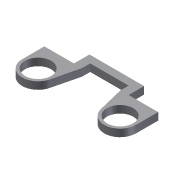
# Autodesk Inventor part: Suporte - Baterias
Saved by Autodesk Inventor 2011 (Build 150239000, 239)
## iProperties
Created: 2011-04-09
Part Number: Suporte - Baterias
Document SubType Name: Modeling
Designer: Milton
Density: 1 g/cm^3
Author: Milton
Autodesk Inventor part; units mm, degrees
ref_plane "YZ Plane" through (0, 0, 0) normal (1, 0, 0) x (0, 1, 0)
ref_plane "XZ Plane" through (0, 0, 0) normal (0, 1, 0) x (-1, 0, 0)
ref_plane "XY Plane" through (0, 0, 0) normal (0, 0, 1) x (1, 0, 0)
sketch "Sketch1" plane through (0, 0, 0) normal (0, 0, 1) x (1, 0, 0)
  line L0 (38.75, 17.7481) -> (-13.25, 17.75)
  circle A0 centre (68.25, -23.2519) radius 17.75
  circle A1 centre (-42.75, -23.2512) radius 17.75
  circle A2 centre (68.25, -23.2519) radius 21.5
  circle A3 centre (-42.75, -23.2512) radius 21.5
  line L1 (49.75, 27.75) -> (-24.25, 27.75)
  line L2 (-24.25, 6.7504) -> (-74.75, 6.7484)
  line L3 (49.75, 27.75) -> (49.75, 6.7488)
  line L4 (38.75, 17.7481) -> (38.75, 6.7503)
  line L5 (-13.25, 17.75) -> (-13.25, 6.7503)
  line L6 (-24.25, 27.75) -> (-24.25, 6.7504)
  line L7 (38.75, 6.7503) -> (47.3695, -28.3757)
  line L8 (-13.25, 6.7503) -> (-21.8695, -28.3751)
  line L9 (-74.75, 6.7503) -> (-74.75, -44.7512)
  line L10 (-42.75, -44.7512) -> (-74.75, -44.7512)
  line L11 (68.25, -44.7519) -> (100.25, -44.7519)
  line L12 (100.25, -44.7519) -> (100.25, 6.7488)
  line L13 (49.75, 6.7488) -> (100.25, 6.7488)
  point P0 (0, 0)
  point P1 (-64.25, -23.2512)
  point P2 (89.75, -23.2512)
  dimension "d6" = 35.5
  dimension "d7" = 35.5
  dimension "d14" = 43
  dimension "d15" = 43
  dimension "d23" = 52
  dimension "d25" = 11
  dimension "d26" = 11
  dimension "d29" = 29.5
  dimension "d30" = 29.5
  dimension "d31" = 32
  dimension "d32" = 32
  constraints: 28 end point, 6 point on circle, 4 centre point, 4 parallel, 4 tangent, 3 perpendicular, 2 coincident, 1 point on line
  measures "d6" diameter of A0
  measures "d7" diameter of A1
  measures "d14" diameter of A2
  measures "d15" diameter of A3
  measures "d23" distance of L0.start L0.end
  measures "d25" distance between parallel lines of L3 L4
  measures "d26" distance between parallel lines of L6 L5
  measures "d29" distance from line of L4 A0.centre
  measures "d30" distance from line of A1.centre L5
  measures "d31" distance from line of L12 A2.centre
  measures "d32" distance from line of A1.centre L9
extrude "Extrusion1" add sketch "Sketch1" along normal blind 10
sketch "Sketch2" plane through (68.25, -44.7519, 0) normal (0, -1, 0) x (1, 0, 0)
  line L0 (32, 0) -> (32, 10) projected
  circle A0 centre (-136.5, 5) radius 4.1
  circle A1 centre (25.5, 5) radius 4.1
  point P0 (-68.25, 0)
  dimension "d33" = 8.2
  dimension "d34" = 8.2
  dimension "d35" = 162
  dimension "d36" = 6.5
  constraints: 2 centre point
  measures "d33" diameter of A0
  measures "d34" diameter of A1
  measures "d35" distance of A0.centre A1.centre
  measures "d36" distance from line of L0 A1.centre
extrude "Extrusion2" cut sketch "Sketch2" against normal through all
body "Solid1"
